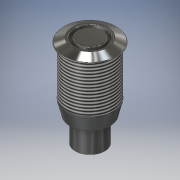
# Autodesk Inventor part: Button_housing
Saved by Autodesk Inventor 2016 (Build 200138000, 138)
## iProperties
Created: 2016-04-10
Part Number: Button_housing
Material: Brass, Soft Yellow
Document SubType Name: Modeling
Designer: agmle
Mass: 41.027 g
Surface Area: 18.0121 cm^2
Volume: 5.12837 cm^3
Density: 8.47 g/cm^3
Appearance: Chrome - Polished
Author: agmle
Autodesk Inventor part; units mm, degrees
ref_plane "YZ Plane" through (0, 0, 0) normal (1, 0, 0) x (0, 1, 0)
ref_plane "XZ Plane" through (0, 0, 0) normal (0, 1, 0) x (-1, 0, 0)
ref_plane "XY Plane" through (0, 0, 0) normal (0, 0, 1) x (1, 0, 0)
sketch "Sketch1" plane through (0, 0, 0) normal (0, 1, 0) x (-1, 0, 0)
  circle A0 centre (0, 0) radius 8
  dimension "d0" = 16
  constraints: 1 centre point, 1 coincident
  measures "d0" diameter of A0
extrude "Extrusion1" add sketch "Sketch1" along normal blind 29.7
sketch "Sketch2" plane through (0, 29.7, 0) normal (0, 1, 0) x (1, 0, 0)
  circle A0 centre (0, 0) radius 9
  dimension "d3" = 18
  constraints: 1 centre point, 1 coincident
  measures "d3" diameter of A0
extrude "Extrusion2" add sketch "Sketch2" along normal blind 1.5
chamfer "Chamfer1" distance 3 distance2 1.25 1 edges at (-9, 31.2, 0) measured on face at (4.3113, 31.2, 2.4985)
sketch "Sketch3" plane through (0, 0, 0) normal (0, -1, 0) x (1, 0, 0)
  circle A0 centre (0, 0) radius 5
  circle A1 centre (0, 0) radius 8 projected
  dimension "d9" = 10
  constraints: 1 centre point, 1 coincident
  measures "d9" diameter of A0
extrude "Extrusion3" cut sketch "Sketch3" against normal blind 8
chamfer "Chamfer2" distance 5 distance2 1.25 1 edges at (8, 8, 0) measured on face at (-7.8964, 15.2333, -1.2833)
fillet "Fillet1" radius 3.175 1 edges at (8, 13, 0)
fillet "Fillet2" radius 0.5 1 edges at (6.75, 8, 0)
thread "Thread1" size "M16x1" class "6g" standard "ISO Metric profile" full length
sketch "Sketch4" plane through (0, 31.2, 0) normal (0, 1, 0) x (1, 0, 0)
  circle A0 centre (0, 0) radius 4.25
  circle A1 centre (0, 0) radius 5.25
  circle A2 centre (0, 0) radius 6 construction
  dimension "d22" = 0.75
  dimension "d23" = 1
  dimension "d25" = 10.5
  constraints: 2 centre point, 2 coincident
  measures "d22" radial gap between concentric circles of A2 A1
  measures "d23" radial gap between concentric circles of A1 A0
  measures "d25" diameter of A1
extrude "Extrusion4" cut sketch "Sketch4" against normal blind 1.5
fillet "Fillet3" radius 0.25 4 edges at (-9, 29.95, 0) (-6, 31.2, 0) (-5.25, 31.2, 0) (-4.25, 31.2, 0)
body "Solid1"
